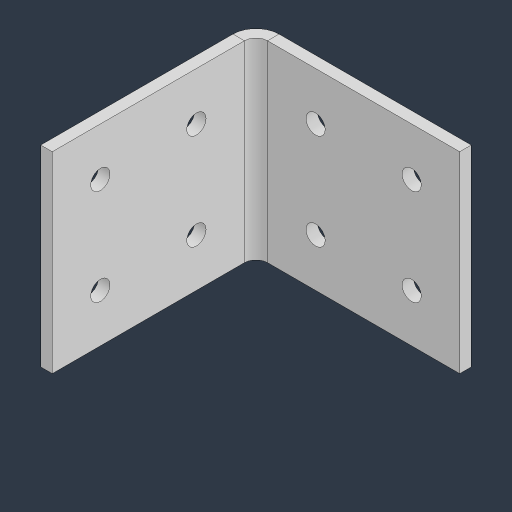
# Autodesk Inventor part: hopper_side_barcket
Saved by Autodesk Inventor 2024.3 (Build 283343000, 343)
## iProperties
Created: 2025-03-08
Part Number: hopper_side_barcket
Material: Generic
Document SubType Name: Sheet Metal
Designer: marcu
Density: 1 g/cm^3
Sheet Metal Rule: Default
Appearance: Default
Author: marcu
Autodesk Inventor part; units mm, degrees
ref_plane "YZ Plane" through (0, 0, 0) normal (1, 0, 0) x (0, 1, 0)
ref_plane "XZ Plane" through (0, 0, 0) normal (0, 1, 0) x (-1, 0, 0)
ref_plane "XY Plane" through (0, 0, 0) normal (0, 0, 1) x (1, 0, 0)
sketch "Sketch1" plane through (0, 0, 0) normal (0, 0, 1) x (1, 0, 0)
  line L0 (25.4, 25.4) -> (-25.4, 25.4)
  line L1 (-25.4, 25.4) -> (-25.4, -25.4)
  line L2 (-25.4, -25.4) -> (25.4, -25.4)
  line L3 (25.4, -25.4) -> (25.4, 25.4)
  line L4 (25.4, 25.4) -> (-25.4, -25.4) construction
  line L5 (-25.4, 25.4) -> (25.4, -25.4) construction
  point P0 (0, 0)
  dimension "d0" = 50.8
  dimension "d1" = 50.8
  measures "d0" distance of L2.end L1.end
  measures "d1" distance of L1.end L0.end
extrude "Plate1" add sketch "Sketch1" along normal blind 3.048
sketch "Sketch2" plane through (-28.448, -25.4, 6.096) normal (-1, 0, 0) x (0, -1, 0)
  line L0 (-50.8, 0) -> (0, 0)
  line L1 (0, 0) -> (0, 50.8)
  line L2 (0, 50.8) -> (-50.8, 50.8)
  line L3 (-50.8, 50.8) -> (-50.8, 0)
  constraints: 6 end point, 1 horizontal, 1 perpendicular, 1 vertical
edge flange "Flange1" height 56.896 angle 90 thickness 3.048 bend radius 3.048 thickness toward (-1, 0, 0) relief tear relief width 3.048 relief depth 1.524 edges at (-25.4, 0, 3.048) wall of the first edge with corners at (-28.448, 25.4, 6.096) (-28.448, -25.4, 6.096) (-28.448, -25.4, 56.896) (-28.448, 25.4, 56.896)
bend "Bend1"
corner "Corner1"
sketch "Sketch3" plane through (-28.448, -25.4, 56.896) normal (1, 0, 0) x (0, 0, -1)
  line L0 (50.8, 0) -> (50.8, 50.8) construction
  line L1 (0, 50.8) -> (50.8, 50.8) construction
  line L2 (0, 50.8) -> (0, 0) construction
  line L3 (0, 0) -> (50.8, 0) construction
  point P0 (56.896, 25.4)
  point P1 (38.1, 38.1)
  point P2 (38.1, 12.7)
  point P3 (12.7, 38.1)
  point P4 (12.7, 12.7)
  dimension "d13" = 12.7
  dimension "d14" = 12.7
  dimension "d17" = 25.4
  dimension "d20" = 25.4
  constraints: 1 horizontal, 1 vertical, 3 other
  measures "d13" distance from line of L0 point (38.1, 38.1)
  measures "d14" distance from line of L1 point (38.1, 38.1)
  measures "d17" distance of point (38.1, 38.1) point (38.1, 12.7)
  measures "d20" distance of point (38.1, 38.1) point (12.7, 38.1)
hole "Hole1" at (-28.448, 12.7, 18.796) at (-28.448, -12.7, 18.796) at (-28.448, 12.7, 44.196) at (-28.448, -12.7, 44.196) direction (-1, 0, 0) diameter 5.1054 end through all clearance for "Flat Head Machine Screw (82)" size "#10" standard "Ansi Unified Screw Threads"
sketch "Sketch4" plane through (0, 0, 3.048) normal (0, 0, 1) x (1, 0, 0)
  line L0 (-25.4, 25.4) -> (25.4, 25.4) construction
  line L1 (-25.4, -25.4) -> (-25.4, 25.4) construction
  line L2 (25.4, -25.4) -> (-25.4, -25.4) construction
  line L3 (25.4, 25.4) -> (25.4, -25.4) construction
  point P0 (0, 0)
  point P1 (-12.7, 12.7)
  point P2 (12.7, 12.7)
  point P3 (-12.7, -12.7)
  point P4 (12.7, -12.7)
  dimension "d30" = 12.7
  dimension "d31" = 12.7
  dimension "d34" = 25.4
  dimension "d37" = 25.4
  constraints: 1 horizontal, 1 vertical, 3 other
  measures "d30" distance from line of L0 point (-12.7, 12.7)
  measures "d31" distance from line of L1 point (-12.7, 12.7)
  measures "d34" distance of point (-12.7, 12.7) point (12.7, 12.7)
  measures "d37" distance of point (-12.7, 12.7) point (-12.7, -12.7)
hole "Hole2" at (-12.7, 12.7, 3.048) at (12.7, 12.7, 3.048) at (-12.7, -12.7, 3.048) at (12.7, -12.7, 3.048) direction (0, 0, -1) diameter 5.1054 end through all clearance for "Flat Head Machine Screw (82)" size "#10" standard "Ansi Unified Screw Threads"
equation "\"d28\" = Thickness"
equation "\"d2\" = Thickness"
equation "\"d3\" = BendReliefWidth"
equation "\"d4\" = BendReliefDepth"
equation "\"d5\" = MinimumRemnant"
equation "\"d6\" = TransitionRadius"
equation "\"d9\" = BendRadius"
equation "\"d10\" = CornerReliefSize"
equation "\"d11\" = GapSize"
equation "\"d12\" = JacobiRadiusSize"
equation "\"BendRadius\" = Thickness"
equation "\"BendReliefWidth\" = Thickness"
equation "\"BendReliefDepth\" = 0.5 * Thickness"
equation "\"CornerReliefSize\" = 4 * Thickness"
equation "\"MinimumRemnant\" = 2 * Thickness"
equation "\"TransitionRadius\" = BendRadius"
equation "\"JacobiRadiusSize\" = BendRadius"
equation "\"GapSize\" = Thickness"
equation "\"Thickness\" = 3.048"
body "Solid1"
